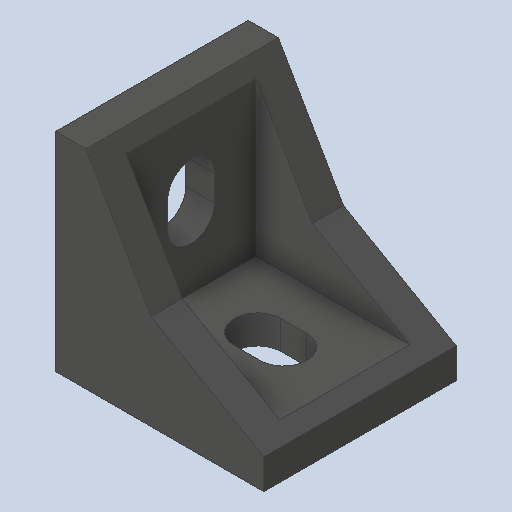
# Autodesk Inventor part: GUS_4501_1
Saved by Autodesk Inventor 2023 (Build 270158000, 158)
## iProperties
Created: 2023-08-22
Part Number: GUS_4501_1
Material: Generic
Catalog Web Link: www.cadenas.de
Description: GUS 4500-Angle
Vendor: ROBOTUNITS
Document SubType Name: Modeling
Designer: psAdmin
Manufacturer: ROBOTUNITS
Mass: 21.5116 g
Surface Area: 82.4481 cm^2
Volume: 21.5116 cm^3
Density: 1 g/cm^3
Appearance: PSOLRGB-91-91-91
Category: PARTsolutions
Company: ROBOTUNITS
PSOL_IDENT_0: {$CADENAS_DATA/23d-libs/robotunits/profil_und_verbindungstechnik/verbindungstechnik_raster_40/parts/
PSOL_IDENT_1: gus_4500.prj},162 {VTYP=3D},{NB=GUS_4501_1},{LINA=GUS_4501_1},{NN=GUS 4500},{DATE=01.02.2021 09:12:1
PSOL_IDENT_2: 1},{GEOMDATE=26.11.2014 16:55:00},{VERSION=},{LINEID=50},{WBVAR=},{WBNUMERIC=}  {NB=GUS_4501_1},{LIN
PSOL_IDENT_3: A=GUS_4501_1},{KT=DUMMY},{ARTIKEL=GUS_4501_1},{M=M8},{NDM=8.000},{KDM=6.647},{VERS=1.000}
NB: GUS_4501_1
NN: GUS 4500
NT: Angle
NBSYN: $ARTIKEL.
LINA: GUS_4501_1
CATALOG: Robotunits
ARTIKEL: GUS_4501_1
M: M8
NDM: 8
KDM: 6.647
VERS: 1
SUPPLIER: ROBOTUNITS
ARTICLENO: GUS_4501_1
BOMINFO: GUS_4501_1
CREATOR: CADENAS GmbH
Title: GUS_4501_1
Author: Cadenas PARTsolutions
Comments: Angle
Autodesk Inventor part; units mm, degrees
sketch "Skizze_1" plane through (0, 0, 0) normal (0, 0, 1) x (1, 0, 0)
  line L0 (0, 0) -> (40, 0)
  line L1 (40, 0) -> (40, 5.8)
  line L2 (40, 5.8) -> (18.3181, 18.3181)
  line L3 (18.3181, 18.3181) -> (5.8, 40)
  line L4 (5.8, 40) -> (0, 40)
  line L5 (0, 40) -> (0, 0)
  constraints: 12 end point
extrude "Extrusion1" add sketch "Skizze_1" along normal mid plane 37
sketch "Skizze_2" plane through (0, 0, 0) normal (0, 0, 1) x (1, 0, 0)
  line L0 (7.5, 7.5) -> (40, 7.5)
  line L1 (40, 7.5) -> (40, 40)
  line L2 (40, 40) -> (7.5, 40)
  line L3 (7.5, 40) -> (7.5, 7.5)
  constraints: 8 end point
extrude "Extrusion2" cut sketch "Skizze_2" along normal mid plane 25
sketch "Skizze_3" plane through (0, 0, 0) normal (0, 1, 0) x (-1, 0, 0)
  arc A0 (-20.3, -4.5) -> (-20.3, 4.5) centre (-20.3, 0) ccw
  line L0 (-20.3, 4.5) -> (-25.3, 4.5)
  arc A1 (-25.3, 4.5) -> (-25.3, -4.5) centre (-25.3, 0) ccw
  line L1 (-25.3, -4.5) -> (-20.3, -4.5)
  constraints: 4 end point, 4 point on circle, 2 centre point
extrude "Extrusion3" cut sketch "Skizze_3" along normal blind 7.5
sketch "Skizze_4" plane through (0, 0, 0) normal (1, 0, 0) x (0, 1, 0)
  arc A0 (20.3, 4.5) -> (20.3, -4.5) centre (20.3, 0) ccw
  line L0 (20.3, -4.5) -> (25.3, -4.5)
  arc A1 (25.3, -4.5) -> (25.3, 4.5) centre (25.3, 0) ccw
  line L1 (25.3, 4.5) -> (20.3, 4.5)
  constraints: 4 end point, 4 point on circle, 2 centre point
extrude "Extrusion4" cut sketch "Skizze_4" along normal blind 7.5
sketch "Skizze_5" plane through (0, 0, 0) normal (1, 0, 0) x (0, 1, 0)
  line L0 (13, 7) -> (13, -7)
  line L1 (13, -7) -> (32, -7)
  line L2 (32, -7) -> (32, 7)
  line L3 (32, 7) -> (13, 7)
  constraints: 8 end point
extrude "Extrusion5" cut sketch "Skizze_5" along normal blind 2
sketch "Skizze_6" plane through (0, 0, 0) normal (0, 1, 0) x (-1, 0, 0)
  line L0 (-13, 7) -> (-32, 7)
  line L1 (-32, 7) -> (-32, -7)
  line L2 (-32, -7) -> (-13, -7)
  line L3 (-13, -7) -> (-13, 7)
  constraints: 8 end point
extrude "Extrusion6" cut sketch "Skizze_6" along normal blind 2
ref_plane "GUS_4500_1_XY" through (7.5, 20, 0) normal (1, 0, 0) x (0, 0, -1)
ref_plane "GUS_4500_1_YZ" through (7.5, 20, 0) normal (0, 0, -1) x (0, 1, 0)
ref_plane "GUS_4500_1_ZX" through (7.5, 20, 0) normal (0, 1, 0) x (1, 0, 0)
ref_plane "GUS_4500_12_XY" through (7.5, 25, 0) normal (1, 0, 0) x (0, 0, -1)
ref_plane "GUS_4500_12_YZ" through (7.5, 25, 0) normal (0, 0, -1) x (0, 1, 0)
ref_plane "GUS_4500_12_ZX" through (7.5, 25, 0) normal (0, 1, 0) x (1, 0, 0)
ref_plane "GUS_4500_2_XY" through (25, 7.5, 0) normal (0, 1, 0) x (1, 0, 0)
ref_plane "GUS_4500_2_YZ" through (25, 7.5, 0) normal (1, 0, 0) x (0, 0, -1)
ref_plane "GUS_4500_2_ZX" through (25, 7.5, 0) normal (0, 0, -1) x (0, 1, 0)
ref_plane "GUS_4500_23_XY" through (20, 7.5, 0) normal (0, 1, 0) x (1, 0, 0)
ref_plane "GUS_4500_23_YZ" through (20, 7.5, 0) normal (1, 0, 0) x (0, 0, -1)
ref_plane "GUS_4500_23_ZX" through (20, 7.5, 0) normal (0, 0, -1) x (0, 1, 0)
ref_plane "p1_XY" through (0, 20, -18.5) normal (0, 0, -1) x (0, 1, 0)
ref_plane "p1_YZ" through (0, 20, -18.5) normal (0, 1, 0) x (1, 0, 0)
ref_plane "p1_ZX" through (0, 20, -18.5) normal (1, 0, 0) x (0, 0, -1)
body "Solid1"
